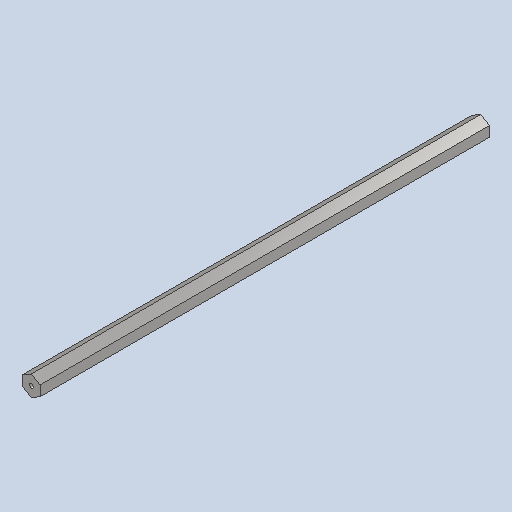
# Autodesk Inventor part: SHAFT,HEX,0.500in,DRIVE,ELEVATOR
Saved by Autodesk Inventor 2025.2 (Build 292293000, 293)
## iProperties
Created: 2025-01-29
Part Number: SHAFT,HEX,0.500in,DRIVE,ELEVATOR
Material: Steel, Alloy
Description: STEP AP214
Document SubType Name: Modeling
Designer: dave.simone
Density: 7.73 g/cm^3
Appearance: Semi-Polished
Mfg Approved By: John.Thibert
Mass: 333.761 g
Surface Area: 174.084 cm^2
Volume: 43.1773 cm^3
ILogicPurgeVersion: 0.0.0.0
OnSaveVersion: 3.5.0.0
OnSaveAssembly: COREAutomationManager
Sending System: SolidWorks 2017
Preprocessor: SwSTEP 2.0
ModelCat: Uncategorized
MaterialName: Steel, Alloy
CN_MASS: 0.33
Title: am-0856 500 Hex Shaft for Modulox REV3.STEP
Revision Number: ANY
Autodesk Inventor part; units mm, degrees
ref_plane "YZ Plane" through (0, 0, 0) normal (1, 0, 0) x (0, 1, 0)
ref_plane "XZ Plane" through (0, 0, 0) normal (0, 1, 0) x (-1, 0, 0)
ref_plane "XY Plane" through (0, 0, 0) normal (0, 0, 1) x (1, 0, 0)
sketch "Sketch1" plane through (0, 0, 0) normal (0, 0, 1) x (1, 0, 0)
  line L0 (6.35, 3.6662) -> (6.35, -3.6662)
  line L1 (6.35, -3.6662) -> (0, -7.3323)
  line L2 (0, -7.3323) -> (-6.35, -3.6662)
  line L3 (-6.35, -3.6662) -> (-6.35, 3.6662)
  line L4 (-6.35, 3.6662) -> (0, 7.3323)
  line L5 (0, 7.3323) -> (6.35, 3.6662)
  circle A0 centre (0, 0) radius 1.4224
  dimension "d0" = 12.7
  dimension "d3" = 2.8448
  constraints: 12 end point, 2 coincident, 1 centre point, 1 vertical, 13 other
  measures "d0" distance between parallel lines of L0 L3
  measures "d3" diameter of A0
extrude "Extrusion1" add sketch "Sketch1" against normal blind 323.85
body "Solid2"
